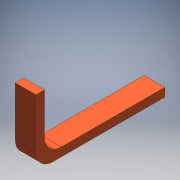
# Autodesk Inventor part: pin
Saved by Autodesk Inventor 2016 (Build 200138000, 138)
## iProperties
Created: 2016-08-01
Part Number: pin
Material: Copper
Document SubType Name: Modeling
Designer: Jonathan
Density: 8.94 g/cm^3
Appearance: Copper - Satin
Author: Jonathan
Autodesk Inventor part; units mm, degrees
ref_plane "YZ Plane" through (0, 0, 0) normal (1, 0, 0) x (0, 1, 0)
ref_plane "XZ Plane" through (0, 0, 0) normal (0, 1, 0) x (-1, 0, 0)
ref_plane "XY Plane" through (0, 0, 0) normal (0, 0, 1) x (1, 0, 0)
sketch "Sketch1" plane through (0, 0, 0) normal (1, 0, 0) x (0, 1, 0)
  line L0 (3.81, 0.254) -> (0.254, 0.254)
  line L1 (0.254, 0.254) -> (0.254, 1.9685)
  line L2 (0.254, 1.9685) -> (0, 1.9685)
  line L3 (0, 1.9685) -> (0, 0)
  line L4 (0, 0) -> (3.81, 0)
  line L5 (3.81, 0) -> (3.81, 0.254)
  dimension "d0" = 0.254
  dimension "d1" = 3.81
  dimension "d2" = 1.7145
  dimension "d3" = 0.254
  constraints: 12 end point, 5 perpendicular, 1 coincident, 1 horizontal
  measures "d0" distance between parallel lines of L3 L1
  measures "d1" distance between parallel lines of L5 L3
  measures "d2" distance between parallel lines of L2 L0
  measures "d3" distance between parallel lines of L4 L0
extrude "Extrusion1" add sketch "Sketch1" along normal mid plane 0.6096
fillet "Fillet1" radius 0.5 2 edges at (0, 0, 0) (0, 0.254, 0.254)
body "Solid1"
